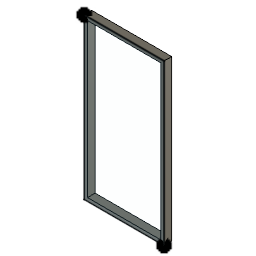
_WIndowPlugOne.25eca7a3-5849-49ac-8090-5e45aaec9fa8 (Autodesk Fusion 360 design; units mm, degrees)
Autodesk Fusion 360 part; units mm, degrees
sketch "Sketch1" plane through (0, 0, 0) normal (0, 0, 1) x (1, 0, 0)
  line L0 (-121.92, 12.192) -> (792.48, 12.192)
  line L1 (792.48, 12.192) -> (792.48, -76.708)
  line L2 (792.48, -76.708) -> (-121.92, -76.708)
  line L3 (-121.92, -76.708) -> (-121.92, 12.192)
  dimension "d1" = 914.4
  dimension "d6" = 88.9
  constraint horizontal L0
  constraint vertical L1
  constraint horizontal L2
  constraint vertical L3
  measures "d1" distance of L0.start L0.end
  measures "d6" distance of L0.start L2.end
extrude "Extrude1" add sketch "Sketch1" along normal blind 38.1
sketch "Sketch2" plane through (0, 0, 38.1) normal (0, 0, 1) x (-1, 0, 0)
  line L0 (121.92, 76.708) -> (-792.48, 76.708)
  line L1 (-792.48, 76.708) -> (-792.48, -12.192)
  line L2 (-792.48, -12.192) -> (121.92, -12.192)
  line L3 (121.92, -12.192) -> (121.92, 76.708)
  line L4 (121.92, -12.192) -> (83.82, -12.192)
  line L5 (83.82, -12.192) -> (83.82, 76.708)
  line L6 (83.82, 76.708) -> (121.92, 76.708)
  line L7 (121.92, 76.708) -> (121.92, -12.192)
  line L8 (-792.48, -12.192) -> (-754.38, -12.192)
  line L9 (-754.38, -12.192) -> (-754.38, 76.708)
  line L10 (-754.38, 76.708) -> (-792.48, 76.708)
  line L11 (-792.48, 76.708) -> (-792.48, -12.192)
  dimension "d9" = 38.1
  dimension "d10" = 38.1
  constraint horizontal L4
  constraint vertical L5
  constraint horizontal L6
  constraint vertical L7
  constraint coincident L0 L5.end
  constraint coincident L2.end L3.start
  constraint horizontal L8
  constraint vertical L9
  constraint horizontal L10
  constraint vertical L11
  constraint coincident L0 L9.end
  constraint coincident L1.end L2.start
  measures "d9" distance of L5 L7
  measures "d10" distance of L9 L11
extrude "Extrude2" add sketch "Sketch2" along normal blind 1752.6 contours L0 L2 L3 L4 L5 L6 L7 | L0 L1 L2 L8 L9 L10 L11
sketch "Sketch3" plane through (0, 0, 1790.7) normal (0, 0, 1) x (-1, 0, 0)
  line L0 (121.92, 76.708) -> (83.82, 76.708)
  line L1 (83.82, 76.708) -> (83.82, -12.192)
  line L2 (83.82, -12.192) -> (121.92, -12.192)
  line L3 (121.92, -12.192) -> (121.92, 76.708)
  line L4 (121.92, 76.708) -> (-792.48, 76.708)
  line L5 (-792.48, 76.708) -> (-792.48, -12.192)
  line L6 (-792.48, -12.192) -> (121.92, -12.192)
  line L7 (121.92, -12.192) -> (121.92, 76.708)
  dimension "d13" = 88.9
  dimension "d14" = 914.4
  constraint horizontal L4
  constraint vertical L5
  constraint horizontal L6
  constraint vertical L7
  constraint coincident L0.start L3.end
  measures "d13" distance of L4 L6
  measures "d14" distance of L5.end L2.end
extrude "Extrude3" add sketch "Sketch3" along normal blind 38.1
sketch "Sketch4" plane through (0, -76.708, 0) normal (0, -1, 0) x (1, 0, 0)
  line L0 (754.38, 1790.7) -> (754.38, 38.1)
  line L1 (754.38, 38.1) -> (-83.82, 38.1)
  line L2 (-83.82, 38.1) -> (-83.82, 1790.7)
  line L3 (-83.82, 1790.7) -> (754.38, 1790.7)
  line L4 (792.48, 0) -> (792.48, 1828.8)
  line L5 (792.48, 1828.8) -> (-121.92, 1828.8)
  line L6 (-121.92, 1828.8) -> (-121.92, 0)
  line L7 (-121.92, 0) -> (792.48, 0)
  line L8 (-121.92, 1828.8) -> (792.48, 1828.8)
  line L9 (792.48, 1828.8) -> (792.48, 0)
  line L10 (792.48, 0) -> (-121.92, 0)
  line L11 (-121.92, 0) -> (-121.92, 1828.8)
  dimension "d17" = 914.4
  dimension "d18" = 1828.8
  constraint horizontal L8
  constraint vertical L9
  constraint horizontal L10
  constraint vertical L11
  constraint coincident L4.start L7.end
  constraint coincident L5.end L6.start
  measures "d17" distance of L5.end L4.end
  measures "d18" distance of L5.end L6.end
equation "d1 = BottomLength / 2"
equation "BottomLength = 6 ft"
equation "TopLength = 6 ft"
equation "RightLength = 6 ft"
equation "LeftLength = 6 ft"
equation "d11 = RightLength - ( ( ( 2 * 1.5 ) / 12 ) * 1 ft )"
equation "d14 = TopLength / 2"
